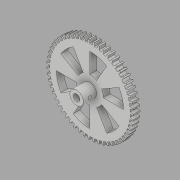
# Autodesk Inventor part: Gear
Saved by Autodesk Inventor 2017 (Build 210142000, 142)
## iProperties
Created: 2017-05-07
Part Number: Gear
Material: Generic
Document SubType Name: Modeling
Designer: zallen
Density: 1 g/cm^3
Appearance: Default
Author: zallen
Autodesk Inventor part; units mm, degrees
ref_plane "YZ Plane" through (0, 0, 0) normal (1, 0, 0) x (0, 1, 0)
ref_plane "XZ Plane" through (0, 0, 0) normal (0, 1, 0) x (-1, 0, 0)
ref_plane "XY Plane" through (0, 0, 0) normal (0, 0, 1) x (1, 0, 0)
sketch "Sketch1" plane through (0, 0, 0) normal (0, 0, 1) x (1, 0, 0)
  circle A0 centre (0, 0) radius 38.1
  dimension "d0" = 76.2
  constraints: 1 centre point, 1 coincident
  measures "d0" diameter of A0
extrude "Extrusion1" add sketch "Sketch1" along normal blind 6.35
sketch "Sketch2" plane through (0, 0, 6.35) normal (0, 0, 1) x (1, 0, 0)
  circle A0 centre (0, 0) radius 6.35
  circle A1 centre (0, 0) radius 3.175
  dimension "d3" = 12.7
  dimension "d4" = 6.35
  constraints: 2 centre point, 2 coincident
  measures "d3" diameter of A0
  measures "d4" diameter of A1
extrude "Extrusion2" add sketch "Sketch2" along normal blind 12.7
sketch "Sketch3" plane through (0, 0, 0) normal (1, 0, 0) x (0, 1, 0)
  circle A0 centre (0, 12.7) radius 1.5875
  line L0 (-38.1, 0) -> (38.1, 0) projected
  point P0 (0, 0)
  dimension "d7" = 3.175
  dimension "d8" = 12.7
  constraints: 1 centre point
  measures "d7" diameter of A0
  measures "d8" distance from line of A0.centre L0
extrude "Extrusion3" cut sketch "Sketch3" along normal through all
sketch "Sketch4" plane through (0, 0, 6.35) normal (0, 0, 1) x (1, 0, 0)
  circle A0 centre (0, 0) radius 38.1 projected
  line L0 (38.0865, 1.016) -> (41.021, 0.6297)
  line L1 (41.021, 0.6297) -> (41.021, -0.6297)
  line L2 (41.021, -0.6297) -> (38.0865, -1.016)
  line L3 (0, 0) -> (37.2139, 0) construction
  line L4 (0, 0) -> (37.2139, 0) construction
  line L5 (40.8254, 4.0505) -> (37.954, 3.3322)
  line L6 (40.6818, 5.3016) -> (40.8254, 4.0505)
  line L7 (37.7224, 5.3509) -> (40.6818, 5.3016)
  line L8 (40.0976, 8.6778) -> (37.3268, 7.6369)
  line L9 (39.8123, 9.9044) -> (40.0976, 8.6778)
  line L10 (36.8665, 9.6161) -> (39.8123, 9.9044)
  line L11 (38.847, 13.192) -> (36.2129, 11.842)
  line L12 (38.4238, 14.3781) -> (38.847, 13.192)
  line L13 (35.5301, 13.7558) -> (38.4238, 14.3781)
  line L14 (37.09, 17.5343) -> (34.627, 15.8928)
  line L15 (36.5344, 18.6644) -> (37.09, 17.5343)
  line L16 (33.7304, 17.7163) -> (36.5344, 18.6644)
  line L17 (34.8495, 21.6479) -> (32.5897, 19.7364)
  line L18 (34.1686, 22.7073) -> (34.8495, 21.6479)
  line L19 (31.4911, 21.4458) -> (34.1686, 22.7073)
  line L20 (32.1546, 25.4794) -> (30.1274, 23.3227)
  line L21 (31.3575, 26.4542) -> (32.1546, 25.4794)
  line L22 (28.8412, 24.8957) -> (31.3575, 26.4542)
  line L23 (29.0406, 28.9786) -> (27.2725, 26.6049)
  line L24 (28.1375, 29.8563) -> (29.0406, 28.9786)
  line L25 (25.8153, 28.0211) -> (28.1375, 29.8563)
  line L26 (25.548, 32.1001) -> (24.062, 29.5403)
  line L27 (24.5508, 32.8691) -> (25.548, 32.1001)
  line L28 (22.4528, 30.7812) -> (24.5508, 32.8691)
  line L29 (21.7223, 34.8031) -> (20.5378, 32.0906)
  line L30 (20.6439, 35.4534) -> (21.7223, 34.8031)
  line L31 (18.7977, 33.14) -> (20.6439, 35.4534)
  line L32 (17.6135, 37.0524) -> (16.7459, 34.2226)
  line L33 (16.468, 37.5756) -> (17.6135, 37.0524)
  line L34 (14.8975, 35.0667) -> (16.468, 37.5756)
  line L35 (13.275, 38.8187) -> (12.7356, 35.9084)
  line L36 (12.0773, 39.2079) -> (13.275, 38.8187)
  line L37 (10.8031, 36.5363) -> (12.0773, 39.2079)
  line L38 (8.7635, 40.0789) -> (8.5594, 37.1261)
  line L39 (7.5293, 40.329) -> (8.7635, 40.0789)
  line L40 (6.5678, 37.5296) -> (7.5293, 40.329)
  line L41 (4.1377, 40.8166) -> (4.2715, 37.8598)
  line L42 (2.883, 40.9244) -> (4.1377, 40.8166)
  line L43 (2.247, 38.0337) -> (2.883, 40.9244)
  line L44 (-0.542, 41.0223) -> (-0.072, 38.0999)
  line L45 (-1.8008, 40.9863) -> (-0.542, 41.0223)
  line L46 (-2.1032, 38.0419) -> (-1.8008, 40.9863)
  line L47 (-5.2146, 40.6931) -> (-4.4146, 37.8434)
  line L48 (-6.4611, 40.5139) -> (-5.2146, 40.6931)
  line L49 (-6.4259, 37.5542) -> (-6.4611, 40.5139)
  line L50 (-9.8193, 39.8334) -> (-8.6997, 37.0935)
  line L51 (-11.0373, 39.5133) -> (-9.8193, 39.8334)
  line L52 (-10.6649, 36.5769) -> (-11.0373, 39.5133)
  line L53 (-14.296, 38.4544) -> (-12.8713, 35.86)
  line L54 (-15.4695, 37.9975) -> (-14.296, 38.4544)
  line L55 (-14.7648, 35.1228) -> (-15.4695, 37.9975)
  line L56 (-18.5863, 36.5742) -> (-16.8751, 34.159)
  line L57 (-19.7001, 35.9865) -> (-18.5863, 36.5742)
  line L58 (-18.6723, 33.2108) -> (-19.7001, 35.9865)
  line L59 (-22.6343, 34.2171) -> (-20.659, 32.0128)
  line L60 (-23.6738, 33.5063) -> (-22.6343, 34.2171)
  line L61 (-22.3363, 30.8658) -> (-23.6738, 33.5063)
  line L62 (-26.3872, 31.4139) -> (-24.1735, 29.4492)
  line L63 (-27.3389, 30.5893) -> (-26.3872, 31.4139)
  line L64 (-25.7092, 28.1185) -> (-27.3389, 30.5893)
  line L65 (-29.7961, 28.2013) -> (-27.3729, 26.5016)
  line L66 (-30.6476, 27.2735) -> (-29.7961, 28.2013)
  line L67 (-28.7468, 25.0046) -> (-30.6476, 27.2735)
  line L68 (-32.8166, 24.6209) -> (-30.2154, 23.2086)
  line L69 (-33.5568, 23.6021) -> (-32.8166, 24.6209)
  line L70 (-31.4098, 21.5647) -> (-33.5568, 23.6021)
  line L71 (-35.4093, 20.7196) -> (-32.664, 19.613)
  line L72 (-36.0285, 19.6231) -> (-35.4093, 20.7196)
  line L73 (-33.6632, 17.8437) -> (-36.0285, 19.6231)
  line L74 (-37.5403, 16.5482) -> (-34.6868, 15.7618)
  line L75 (-38.0305, 15.3883) -> (-37.5403, 16.5482)
  line L76 (-35.4778, 13.8901) -> (-38.0305, 15.3883)
  line L77 (-39.182, 12.1611) -> (-36.2574, 11.705)
  line L78 (-39.5368, 10.9528) -> (-39.182, 12.1611)
  line L79 (-36.8299, 9.7553) -> (-39.5368, 10.9528)
  line L80 (-40.3128, 7.6154) -> (-37.3554, 7.4957)
  line L81 (-40.5276, 6.3746) -> (-40.3128, 7.6154)
  line L82 (-37.7019, 5.4935) -> (-40.5276, 6.3746)
  line L83 (-40.9182, 2.9705) -> (-37.9663, 3.1887)
  line L84 (-40.99, 1.7132) -> (-40.9182, 2.9705)
  line L85 (-38.0823, 1.16) -> (-40.99, 1.7132)
  line L86 (-40.99, -1.7132) -> (-38.0823, -1.16)
  line L87 (-40.9182, -2.9705) -> (-40.99, -1.7132)
  line L88 (-37.9663, -3.1887) -> (-40.9182, -2.9705)
  line L89 (-40.5276, -6.3746) -> (-37.7019, -5.4935)
  line L90 (-40.3128, -7.6154) -> (-40.5276, -6.3746)
  line L91 (-37.3554, -7.4957) -> (-40.3128, -7.6154)
  line L92 (-39.5368, -10.9528) -> (-36.8299, -9.7553)
  line L93 (-39.182, -12.1611) -> (-39.5368, -10.9528)
  line L94 (-36.2574, -11.705) -> (-39.182, -12.1611)
  line L95 (-38.0305, -15.3883) -> (-35.4778, -13.8901)
  line L96 (-37.5403, -16.5482) -> (-38.0305, -15.3883)
  line L97 (-34.6868, -15.7618) -> (-37.5403, -16.5482)
  line L98 (-36.0285, -19.6231) -> (-33.6632, -17.8437)
  line L99 (-35.4093, -20.7196) -> (-36.0285, -19.6231)
  line L100 (-32.664, -19.613) -> (-35.4093, -20.7196)
  line L101 (-33.5568, -23.6021) -> (-31.4098, -21.5647)
  line L102 (-32.8166, -24.6209) -> (-33.5568, -23.6021)
  line L103 (-30.2154, -23.2086) -> (-32.8166, -24.6209)
  line L104 (-30.6476, -27.2735) -> (-28.7468, -25.0046)
  line L105 (-29.7961, -28.2013) -> (-30.6476, -27.2735)
  line L106 (-27.3729, -26.5016) -> (-29.7961, -28.2013)
  line L107 (-27.3389, -30.5893) -> (-25.7092, -28.1185)
  line L108 (-26.3872, -31.4139) -> (-27.3389, -30.5893)
  line L109 (-24.1735, -29.4492) -> (-26.3872, -31.4139)
  line L110 (-23.6738, -33.5063) -> (-22.3363, -30.8658)
  line L111 (-22.6343, -34.2171) -> (-23.6738, -33.5063)
  line L112 (-20.659, -32.0128) -> (-22.6343, -34.2171)
  line L113 (-19.7001, -35.9865) -> (-18.6723, -33.2108)
  line L114 (-18.5863, -36.5742) -> (-19.7001, -35.9865)
  line L115 (-16.8751, -34.159) -> (-18.5863, -36.5742)
  line L116 (-15.4695, -37.9975) -> (-14.7648, -35.1228)
  line L117 (-14.296, -38.4544) -> (-15.4695, -37.9975)
  line L118 (-12.8713, -35.86) -> (-14.296, -38.4544)
  line L119 (-11.0373, -39.5133) -> (-10.6649, -36.5769)
  line L120 (-9.8193, -39.8334) -> (-11.0373, -39.5133)
  line L121 (-8.6997, -37.0935) -> (-9.8193, -39.8334)
  line L122 (-6.4611, -40.5139) -> (-6.4259, -37.5542)
  line L123 (-5.2146, -40.6931) -> (-6.4611, -40.5139)
  line L124 (-4.4146, -37.8434) -> (-5.2146, -40.6931)
  line L125 (-1.8008, -40.9863) -> (-2.1032, -38.0419)
  line L126 (-0.542, -41.0223) -> (-1.8008, -40.9863)
  line L127 (-0.072, -38.0999) -> (-0.542, -41.0223)
  line L128 (2.883, -40.9244) -> (2.247, -38.0337)
  line L129 (4.1377, -40.8166) -> (2.883, -40.9244)
  line L130 (4.2715, -37.8598) -> (4.1377, -40.8166)
  line L131 (7.5293, -40.329) -> (6.5678, -37.5296)
  line L132 (8.7635, -40.0789) -> (7.5293, -40.329)
  line L133 (8.5594, -37.1261) -> (8.7635, -40.0789)
  line L134 (12.0773, -39.2079) -> (10.8031, -36.5363)
  line L135 (13.275, -38.8187) -> (12.0773, -39.2079)
  line L136 (12.7356, -35.9084) -> (13.275, -38.8187)
  line L137 (16.468, -37.5756) -> (14.8975, -35.0667)
  line L138 (17.6135, -37.0524) -> (16.468, -37.5756)
  line L139 (16.7459, -34.2226) -> (17.6135, -37.0524)
  line L140 (20.6439, -35.4534) -> (18.7977, -33.14)
  line L141 (21.7223, -34.8031) -> (20.6439, -35.4534)
  line L142 (20.5378, -32.0906) -> (21.7223, -34.8031)
  line L143 (24.5508, -32.8691) -> (22.4528, -30.7812)
  line L144 (25.548, -32.1001) -> (24.5508, -32.8691)
  line L145 (24.062, -29.5403) -> (25.548, -32.1001)
  line L146 (28.1375, -29.8563) -> (25.8153, -28.0211)
  line L147 (29.0406, -28.9786) -> (28.1375, -29.8563)
  line L148 (27.2725, -26.6049) -> (29.0406, -28.9786)
  line L149 (31.3575, -26.4542) -> (28.8412, -24.8957)
  line L150 (32.1546, -25.4794) -> (31.3575, -26.4542)
  line L151 (30.1274, -23.3227) -> (32.1546, -25.4794)
  line L152 (34.1686, -22.7073) -> (31.4911, -21.4458)
  line L153 (34.8495, -21.6479) -> (34.1686, -22.7073)
  line L154 (32.5897, -19.7364) -> (34.8495, -21.6479)
  line L155 (36.5344, -18.6644) -> (33.7304, -17.7163)
  line L156 (37.09, -17.5343) -> (36.5344, -18.6644)
  line L157 (34.627, -15.8928) -> (37.09, -17.5343)
  line L158 (38.4238, -14.3781) -> (35.5301, -13.7558)
  line L159 (38.847, -13.192) -> (38.4238, -14.3781)
  line L160 (36.2129, -11.842) -> (38.847, -13.192)
  line L161 (39.8123, -9.9044) -> (36.8665, -9.6161)
  line L162 (40.0976, -8.6778) -> (39.8123, -9.9044)
  line L163 (37.3268, -7.6369) -> (40.0976, -8.6778)
  line L164 (40.6818, -5.3016) -> (37.7224, -5.3509)
  line L165 (40.8254, -4.0505) -> (40.6818, -5.3016)
  line L166 (37.954, -3.3322) -> (40.8254, -4.0505)
  circle A1 centre (0, 0) radius 38.1
  line L167 (38.0865, -1.016) -> (38.0865, 1.016)
  dimension "d11" = 0
  dimension "d13" = 1.016
  dimension "d14" = 41.021
  dimension "d17" = 360
  dimension "d19" = 15
  constraints: 336 end point, 2 point on circle, 2 vertical, 1 centre point, 1 coincident, 1 collinear, 1 concentric, 1 horizontal, 1 point on line, 387 other
  measures "d11" distance between parallel lines of L3 L4
  measures "d13" distance from line of L3 L0.start
  measures "d14" distance from line of point (0, 0) L1
  measures "d19" angle of L2 L0
extrude "Extrusion4" add sketch "Sketch4" against normal blind 6.35 contours A0 L167 | A0 L0 L1 L2 picked at (38.089, -0.2258)
pattern_circular "Circular Pattern1" count 55 over 360 about axis through (0, 0, 0) along (0, 0, 1) of "Extrusion4"
sketch "Sketch5" plane through (0, 0, 0) normal (0, 0, -1) x (-1, 0, 0)
  circle A0 centre (0, 0) radius 6.35
  circle A1 centre (0, 0) radius 3.175
  dimension "d25" = 12.7
  dimension "d26" = 6.35
  constraints: 2 centre point, 2 coincident
  measures "d25" diameter of A0
  measures "d26" diameter of A1
extrude "Extrusion5" add sketch "Sketch5" along normal blind 6.35
sketch "Sketch7" plane through (0, 0, 6.35) normal (0, 0, 1) x (1, 0, 0)
  line L0 (-27.4963, 15.875) -> (-10.9985, 6.35)
  line L1 (-15.875, 27.4963) -> (-6.35, 10.9985)
  arc A0 (-15.875, 27.4963) -> (-27.4963, 15.875) centre (0, 0) ccw
  line L2 (-27.4963, 15.875) -> (0, 0) construction
  line L3 (-15.875, 27.4963) -> (0, 0) construction
  arc A1 (-6.35, 10.9985) -> (-10.9985, 6.35) centre (0, 0) ccw
  line L4 (0, 0) -> (-41.5589, 0) construction
  line L5 (-31.75, 0) -> (-12.7, 0)
  arc A2 (-31.75, 0) -> (-27.4963, -15.875) centre (0, 0) ccw
  line L6 (-27.4963, -15.875) -> (-10.9985, -6.35)
  arc A3 (-12.7, 0) -> (-10.9985, -6.35) centre (0, 0) ccw
  line L7 (-15.875, -27.4963) -> (-6.35, -10.9985)
  arc A4 (-15.875, -27.4963) -> (0, -31.75) centre (0, 0) ccw
  line L8 (0, -31.75) -> (0, -12.7)
  arc A5 (-6.35, -10.9985) -> (0, -12.7) centre (0, 0) ccw
  line L9 (15.875, -27.4963) -> (6.35, -10.9985)
  arc A6 (15.875, -27.4963) -> (27.4963, -15.875) centre (0, 0) ccw
  line L10 (27.4963, -15.875) -> (10.9985, -6.35)
  arc A7 (6.35, -10.9985) -> (10.9985, -6.35) centre (0, 0) ccw
  line L11 (31.75, 0) -> (12.7, 0)
  arc A8 (31.75, 0) -> (27.4963, 15.875) centre (0, 0) ccw
  line L12 (27.4963, 15.875) -> (10.9985, 6.35)
  arc A9 (12.7, 0) -> (10.9985, 6.35) centre (0, 0) ccw
  line L13 (15.875, 27.4963) -> (6.35, 10.9985)
  arc A10 (15.875, 27.4963) -> (0, 31.75) centre (0, 0) ccw
  line L14 (0, 31.75) -> (0, 12.7)
  arc A11 (6.35, 10.9985) -> (0, 12.7) centre (0, 0) ccw
  dimension "d40" = 30
  dimension "d45" = 31.75
  dimension "d48" = 30
  dimension "d49" = 12.7
  dimension "d53" = 360
  constraints: 30 end point, 24 point on circle, 12 centre point, 2 coincident, 2 collinear, 1 horizontal, 61 other
  measures "d40" angle of L1 L0
  measures "d45" radius of A0
  measures "d48" angle of L4 L0
  measures "d49" radius of A1
extrude "Extrusion7" cut sketch "Sketch7" against normal blind 6.35
body "Solid1"
